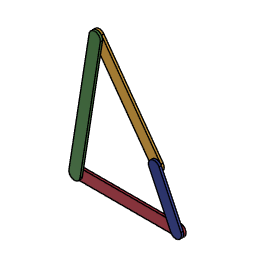
Ande_karthik_msd_q1 v1 (Autodesk Fusion 360 design; units mm, degrees)
Autodesk Fusion 360 part; units mm, degrees
sketch "Sketch1" plane through (0, 0, 0) normal (0, 1, 0) x (1, 0, 0)
  line L0 (0, -10) -> (90, -10)
  arc A0 (90, -10) -> (90, 10) centre (90, 0) ccw
  line L1 (90, 10) -> (0, 10)
  arc A1 (0, 10) -> (0, -10) centre (0, 0) ccw
  line L2 (0, 0) -> (90, 0) construction
  line L3 (0, 24.557) -> (180, 24.557)
  arc A2 (180, 24.557) -> (180, 44.557) centre (180, 34.557) ccw
  line L4 (180, 44.557) -> (0, 44.557)
  arc A3 (0, 44.557) -> (0, 24.557) centre (0, 34.557) ccw
  line L5 (0, 34.557) -> (180, 34.557) construction
  line L6 (0, 70) -> (180, 70)
  arc A4 (180, 70) -> (180, 90) centre (180, 80) ccw
  line L7 (180, 90) -> (0, 90)
  arc A5 (0, 90) -> (0, 70) centre (0, 80) ccw
  line L8 (0, 80) -> (180, 80) construction
  line L9 (0, 120) -> (230, 120)
  arc A6 (230, 120) -> (230, 140) centre (230, 130) ccw
  line L10 (230, 140) -> (0, 140)
  arc A7 (0, 140) -> (0, 120) centre (0, 130) ccw
  line L11 (0, 130) -> (230, 130) construction
  dimension "d1" = 20
  constraint tangent L0 A0
  constraint tangent A0 L1
  constraint parallel L0 L1
  constraint tangent L1 A1
  constraint tangent L0 A1
  constraint horizontal L2
  constraint coincident A1.centre L2.start
  constraint tangent L3 A2
  constraint tangent A2 L4
  constraint parallel L3 L4
  constraint tangent L4 A3
  constraint tangent L3 A3
  constraint parallel L1 L5
  constraint tangent L6 A4
  constraint tangent A4 L7
  constraint parallel L6 L7
  constraint tangent L7 A5
  constraint tangent L6 A5
  constraint horizontal L8
  constraint tangent L9 A6
  constraint tangent A6 L10
  constraint parallel L9 L10
  constraint tangent L10 A7
  constraint tangent L9 A7
  constraint parallel L7 L11
  measures "d1" diameter of A2
extrude "Extrude1" add sketch "Sketch1" along normal blind 4 makes body 1 at (120, 0, -31.2236) makes body 2 at (120, 0, -76.6667) makes body 3 at (60, 0, 3.3333) makes body 4 at (76.6667, 0, -126.6667) in component "Component"
copy_body "Body->Comp1" bodies 1 removing the originals makes body 5 in component "Component'"
copy_body "Body->Comp2" bodies 2 removing the originals makes body 6 in component "Component''"
copy_body "Body->Comp3" bodies 3 removing the originals makes body 7 in component "Component'''"
copy_body "Body->Comp4" bodies 4 removing the originals makes body 8 in component "Component''''"
component "Component" placed x (1, 0, 0) y (0, 1, 0) z (0, 0, 1) at (0, 0, 0)
component "Component'" placed x (1, 0, 0) y (0, 1, 0) z (0, 0, 1) at (0, 0, 0) in component "Component"
component "Component''" placed x (0.679987, 0, -0.733224) y (0, 1, 0) z (0.733224, 0, 0.679987) at (119.0195, 0, 241.78) in component "Component"
component "Component'''" placed x (0.030659, 0, 0.99953) y (0, -1, 0) z (0.99953, 0, -0.030659) at (180, 0, -34.557) in component "Component"
component "Component''''" placed x (0.262442, 0, 0.964948) y (0, -1, 0) z (0.964948, 0, -0.262442) at (125.4432, 0, -68.6744) in component "Component"
